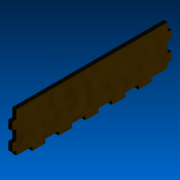
# Autodesk Inventor part: devant
Saved by Autodesk Inventor 2013 SP2 (Build 170200200, 200)
## iProperties
Created: 2015-09-15
Part Number: devant
Material: Generic
Document SubType Name: Modeling
Designer: jeanfrancois
Density: 1 g/cm^3
Author: jeanfrancois
Autodesk Inventor part; units mm, degrees
ref_plane "YZ Plane" through (0, 0, 0) normal (1, 0, 0) x (0, 1, 0)
ref_plane "XZ Plane" through (0, 0, 0) normal (0, 1, 0) x (-1, 0, 0)
ref_plane "XY Plane" through (0, 0, 0) normal (0, 0, 1) x (1, 0, 0)
sketch "Esquisse1" plane through (0, 0, 0) normal (1, 0, 0) x (0, 1, 0)
  line L0 (16.0212, -16.7046) -> (16.0212, -13.7046)
  line L1 (6.0212, -16.7046) -> (16.0212, -16.7046)
  line L2 (6.0212, -16.7046) -> (6.0212, -13.7046)
  line L3 (-3.9788, -16.7046) -> (-3.9788, -13.7046)
  line L4 (-13.9788, -16.7046) -> (-3.9788, -16.7046)
  line L5 (-13.9788, -16.7046) -> (-13.9788, -13.7046)
  line L6 (-25.9788, 9.7954) -> (-25.9788, 16.2954)
  line L7 (-25.9788, -13.7046) -> (-13.9788, -13.7046)
  line L8 (-25.9788, -13.7046) -> (-25.9788, -10.2046)
  line L9 (-25.9788, -4.2046) -> (-25.9788, 3.7954)
  line L10 (-28.9788, -10.2046) -> (-28.9788, -4.2046)
  line L11 (-25.9788, -10.2046) -> (-28.9788, -10.2046)
  line L12 (-25.9788, -4.2046) -> (-28.9788, -4.2046)
  line L13 (-28.9788, 3.7954) -> (-28.9788, 9.7954)
  line L14 (-25.9788, 3.7954) -> (-28.9788, 3.7954)
  line L15 (-25.9788, 9.7954) -> (-28.9788, 9.7954)
  line L16 (91.0212, 3.7954) -> (91.0212, 9.7954)
  line L17 (88.0212, 9.7954) -> (88.0212, 16.2954)
  line L18 (88.0212, 3.7954) -> (91.0212, 3.7954)
  line L19 (88.0212, -4.2046) -> (88.0212, 3.7954)
  line L20 (88.0212, -4.2046) -> (91.0212, -4.2046)
  line L21 (91.0212, -10.2046) -> (91.0212, -4.2046)
  line L22 (88.0212, -10.2046) -> (91.0212, -10.2046)
  line L23 (88.0212, -13.7046) -> (88.0212, -10.2046)
  line L24 (76.0212, -13.7046) -> (88.0212, -13.7046)
  line L25 (76.0212, -16.7046) -> (76.0212, -13.7046)
  line L26 (66.0212, -16.7046) -> (76.0212, -16.7046)
  line L27 (66.0212, -16.7046) -> (66.0212, -13.7046)
  line L28 (56.0212, -13.7046) -> (66.0212, -13.7046)
  line L29 (56.0212, -16.7046) -> (56.0212, -13.7046)
  line L30 (46.0212, -16.7046) -> (46.0212, -13.7046)
  line L31 (46.0212, -16.7046) -> (56.0212, -16.7046)
  line L32 (36.0212, -13.7046) -> (46.0212, -13.7046)
  line L33 (36.0212, -16.7046) -> (36.0212, -13.7046)
  line L34 (26.0212, -16.7046) -> (26.0212, -13.7046)
  line L35 (26.0212, -16.7046) -> (36.0212, -16.7046)
  line L36 (16.0212, -13.7046) -> (26.0212, -13.7046)
  line L37 (-3.9788, -13.7046) -> (6.0212, -13.7046)
  line L38 (-25.9788, 16.2954) -> (88.0212, 16.2954)
  line L39 (88.0212, 9.7954) -> (91.0212, 9.7954)
  point P0 (0, 0)
  constraints: 80 end point
extrude "Extrusion1" add sketch "Esquisse1" along normal blind 3
